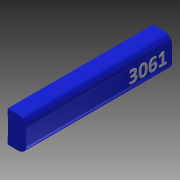
# Autodesk Inventor part: Bumper Cover Part1 (26x28 robot)
Saved by Autodesk Inventor 2013 (Build 170138000, 138)
## iProperties
Created: 2013-01-06
Part Number: Bumper Cover Part1 (26x28 robot)
Material: Generic
Document SubType Name: Modeling
Designer: Moses
Density: 1 g/cm^3
Mass: 433.452 g
Surface Area: 5427.61 cm^2
Volume: 433.452 cm^3
Author: Moses
Autodesk Inventor part; units mm, degrees
ref_plane "YZ Plane" through (0, 0, 0) normal (1, 0, 0) x (0, 1, 0)
ref_plane "XZ Plane" through (0, 0, 0) normal (0, 1, 0) x (-1, 0, 0)
ref_plane "XY Plane" through (0, 0, 0) normal (0, 0, 1) x (1, 0, 0)
sketch "Sketch1" plane through (0, 0, 0) normal (0, 0, 1) x (1, 0, 0)
  line L0 (-6.35, 63.5) -> (-6.35, -63.5) construction
  line L1 (6.35, 63.5) -> (-6.35, 63.5) construction
  line L2 (-6.35, -63.5) -> (6.35, -63.5) construction
  circle A0 centre (38.1, -31.75) radius 31.75 construction
  circle A1 centre (38.1, 31.75) radius 31.75 construction
  line L3 (6.35, 63.5) -> (38.1, 63.5) construction
  line L4 (69.85, 31.75) -> (69.85, -31.75) construction
  line L5 (6.35, -63.5) -> (38.1, -63.5) construction
  line L6 (38.1, 65.0875) -> (-7.9375, 65.0875)
  line L7 (-7.9375, -65.0875) -> (38.1, -65.0875)
  arc A2 (38.1, -65.0875) -> (71.4375, -31.75) centre (38.1, -31.75) ccw
  arc A3 (71.4375, 31.75) -> (38.1, 65.0875) centre (38.1, 31.75) ccw
  line L8 (71.4375, 31.75) -> (71.4375, -31.75)
  line L9 (38.1, 65.0875) -> (38.1, 63.5) construction
  arc A4 (69.85, 31.75) -> (38.1, 63.5) centre (38.1, 31.75) ccw
  arc A5 (38.1, -63.5) -> (69.85, -31.75) centre (38.1, -31.75) ccw
  line L10 (38.1, 63.5) -> (-6.35, 63.5)
  line L11 (38.1, -63.5) -> (-6.35, -63.5)
  line L12 (69.85, 31.75) -> (69.85, -31.75)
  line L13 (-6.35, 63.5) -> (-6.35, 38.1)
  line L14 (-6.35, 38.1) -> (-7.9375, 38.1)
  line L15 (-7.9375, 38.1) -> (-7.9375, 65.0875)
  line L16 (-7.9375, -65.0875) -> (-7.9375, -38.1)
  line L17 (-7.9375, -38.1) -> (-6.35, -38.1)
  line L18 (-6.35, -63.5) -> (-6.35, -38.1)
  line L19 (-6.35, 38.1) -> (-6.35, -38.1)
  point P0 (0, 0)
  point P1 (38.1, 64.2937)
  dimension "d3" = 25.4
  dimension "d5" = 1.5875
  dimension "d6" = 1.5875
  dimension "d7" = 25.4
  dimension "d9" = 1.5875
  constraints: 34 end point, 14 tangent, 12 point on circle, 6 perpendicular, 4 centre point, 3 collinear, 3 parallel, 2 coincident, 2 point on line, 1 concentric, 1 midpoint, 1 vertical
  measures "d3" distance of L0.start L13.end
  measures "d5" distance between parallel lines of L0 L15
  measures "d6" distance between parallel lines of L0 L16
  measures "d7" distance of L0.end L17.end
  measures "d9" distance of L6.start L3.end
extrude "Extrusion1" add sketch "Sketch1" along normal blind 1.5875
extrude "Extrusion2" add sketch "Sketch1" against normal blind 606.425 contours A3 L8 A2 L7 L16 L17 L18 L11 A5 L12 A4 L10 L13 L14 L15 L6
sketch "Sketch2" plane through (0, 0, -606.425) normal (0, 0, -1) x (-1, 0, 0)
  line L0 (-38.1, 63.5) -> (6.35, 63.5) projected
  line L1 (6.35, 63.5) -> (6.35, 38.1) projected
  line L2 (6.35, 38.1) -> (7.9375, 38.1) projected
  line L3 (7.9375, 38.1) -> (7.9375, 65.0875) projected
  line L4 (7.9375, 65.0875) -> (-38.1, 65.0875) projected
  arc A0 (-38.1, 65.0875) -> (-71.4375, 31.75) centre (-38.1, 31.75) ccw projected
  line L5 (-71.4375, 31.75) -> (-71.4375, -31.75) projected
  arc A1 (-71.4375, -31.75) -> (-38.1, -65.0875) centre (-38.1, -31.75) ccw projected
  line L6 (-38.1, -65.0875) -> (7.9375, -65.0875) projected
  line L7 (7.9375, -65.0875) -> (7.9375, -38.1) projected
  line L8 (7.9375, -38.1) -> (6.35, -38.1) projected
  line L9 (6.35, -38.1) -> (6.35, -63.5) projected
  line L10 (6.35, -63.5) -> (-38.1, -63.5) projected
  arc A2 (-69.85, -31.75) -> (-38.1, -63.5) centre (-38.1, -31.75) ccw projected
  line L11 (-69.85, -31.75) -> (-69.85, 31.75) projected
  arc A3 (-38.1, 63.5) -> (-69.85, 31.75) centre (-38.1, 31.75) ccw projected
  line L12 (6.35, 38.1) -> (6.35, -38.1)
  point P0 (0, 0)
  constraints: 2 end point, 1 parallel
extrude "Extrusion3" add sketch "Sketch2" along normal blind 1.5875
sketch "Sketch3" plane through (71.4375, -31.75, 1.5875) normal (1, 0, 0) x (0, 0, -1)
  line L0 (0, 0) -> (0, 63.5) projected
  line L1 (609.6, 63.5) -> (609.6, 0) projected
  line L2 (431.8, 63.5) -> (584.2, 63.5) construction
  line L3 (584.2, 63.5) -> (584.2, 0) construction
  line L4 (584.2, 0) -> (431.8, 0) construction
  line L5 (431.8, 0) -> (431.8, 63.5) construction
  line L6 (609.6, 31.75) -> (0, 31.75) construction
  spline S0 degree 2 poles (464.0687, 21.2561) (464.0687, 17.4878) (461.1591, 11.6208) (456.0075, 7.614) (448.8049, 5.563) (444.5596, 5.563) knots 0 0 0 1 2 3 4 4 4
  spline S1 degree 2 poles (444.5596, 5.563) (441.9839, 5.563) (437.4524, 6.3262) (433.9703, 7.3755) (431.6808, 8.568) (431.013, 9.1881) (430.6314, 9.999) (430.3452, 11.0484) (430.2498, 12.6225) (430.2498, 13.7673) knots 0 0 0 1 2 3 4 5 6 7 8 8 8
  spline S2 degree 2 poles (430.2498, 13.7673) (430.2498, 15.6753) (430.8699, 17.1062) (431.49, 17.1062) knots 0 0 0 1 2 2 2
  spline S3 degree 2 poles (431.49, 17.1062) (431.8716, 17.1062) (433.8272, 16.0569) (436.7846, 14.8167) (440.7914, 13.7673) (443.3194, 13.7673) knots 0 0 0 1 2 3 4 4 4
  spline S4 degree 2 poles (443.3194, 13.7673) (445.4659, 13.7673) (448.7572, 14.769) (451.0468, 16.6293) (452.1915, 19.2527) (452.1915, 20.8268) knots 0 0 0 1 2 3 4 4 4
  spline S5 degree 2 poles (452.1915, 20.8268) (452.1915, 22.5917) (450.8083, 25.406) (448.1371, 27.4093) (444.0349, 28.5064) (441.2207, 28.5064) knots 0 0 0 1 2 3 4 4 4
  line L7 (441.2207, 28.5064) -> (436.8323, 28.5064)
  spline S6 degree 2 poles (436.8323, 28.5064) (436.3553, 28.5064) (435.6398, 28.7926) (435.1628, 29.6512) (434.972, 31.1776) (434.972, 32.3701) knots 0 0 0 1 2 3 4 4 4
  spline S7 degree 2 poles (434.972, 32.3701) (434.972, 33.5149) (435.1628, 34.9459) (435.5921, 35.7091) (436.2599, 36.043) (436.7369, 36.043) knots 0 0 0 1 2 3 4 4 4
  line L8 (436.7369, 36.043) -> (441.173, 36.043)
  spline S8 degree 2 poles (441.173, 36.043) (443.4625, 36.043) (446.9923, 37.0923) (449.3773, 39.048) (450.6175, 41.8146) (450.6175, 43.5318) knots 0 0 0 1 2 3 4 4 4
  spline S9 degree 2 poles (450.6175, 43.5318) (450.6175, 44.8197) (449.7589, 47.1092) (448.0894, 48.7787) (445.4182, 49.7804) (443.6056, 49.7804) knots 0 0 0 1 2 3 4 4 4
  spline S10 degree 2 poles (443.6056, 49.7804) (441.5546, 49.7804) (437.9771, 48.5879) (435.1151, 47.1092) (433.1117, 45.8691) (432.6347, 45.8691) knots 0 0 0 1 2 3 4 4 4
  spline S11 degree 2 poles (432.6347, 45.8691) (432.3485, 45.8691) (431.8716, 46.1553) (431.5377, 46.9185) (431.3946, 48.3971) (431.3946, 49.5896) knots 0 0 0 1 2 3 4 4 4
  spline S12 degree 2 poles (431.3946, 49.5896) (431.3946, 50.5436) (431.49, 51.8315) (431.7285, 52.6901) (432.0623, 53.3102) (432.8255, 54.0734) (435.2582, 55.5521) (438.9311, 56.9831) (443.7487, 57.937) (446.563, 57.937) knots 0 0 0 1 2 3 4 5 6 7 8 8 8
  spline S13 degree 2 poles (446.563, 57.937) (450.2359, 57.937) (455.9121, 56.2199) (459.7758, 52.9763) (461.7792, 48.254) (461.7792, 45.249) knots 0 0 0 1 2 3 4 4 4
  spline S14 degree 2 poles (461.7792, 45.249) (461.7792, 42.9594) (460.5867, 39.0003) (458.3448, 35.8522) (454.9104, 33.658) (452.7162, 33.1333) knots 0 0 0 1 2 3 4 4 4
  line L9 (452.7162, 33.1333) -> (452.7162, 32.9902)
  spline S15 degree 2 poles (452.7162, 32.9902) (455.3397, 32.704) (459.585, 30.6052) (462.4946, 27.5047) (464.0687, 23.5457) (464.0687, 21.2561) knots 0 0 0 1 2 3 4 4 4
  spline S16 degree 2 poles (505.8535, 31.9408) (505.8535, 25.883) (503.8978, 16.1046) (499.4618, 9.2358) (492.4023, 5.563) (487.2984, 5.563) knots 0 0 0 1 2 3 4 4 4
  spline S17 degree 2 poles (487.2984, 5.563) (482.0992, 5.563) (475.2781, 9.1404) (471.3191, 15.8184) (469.6973, 25.4537) (469.6973, 31.5592) knots 0 0 0 1 2 3 4 4 4
  spline S18 degree 2 poles (469.6973, 31.5592) (469.6973, 37.5693) (471.7007, 47.3954) (476.089, 54.2642) (483.1962, 57.937) (488.2524, 57.937) knots 0 0 0 1 2 3 4 4 4
  spline S19 degree 2 poles (488.2524, 57.937) (493.4516, 57.937) (500.3204, 54.3596) (504.2794, 47.6816) (505.8535, 38.0463) (505.8535, 31.9408) knots 0 0 0 1 2 3 4 4 4
  spline S20 degree 2 poles (495.5027, 31.4638) (495.5027, 35.0413) (495.1211, 40.5744) (494.3102, 44.6289) (493.07, 47.4431) (491.3529, 49.1126) (489.1587, 49.8281) (487.8231, 49.8281) knots 0 0 0 1 2 3 4 5 6 6 6
  spline S21 degree 2 poles (487.8231, 49.8281) (485.5335, 49.8281) (482.5285, 47.5862) (480.7636, 43.1502) (480.0481, 36.4723) (480.0481, 32.0839) knots 0 0 0 1 2 3 4 4 4
  spline S22 degree 2 poles (480.0481, 32.0839) (480.0481, 26.6462) (480.9067, 19.5866) (482.7669, 15.3891) (485.6289, 13.7196) (487.68, 13.7196) knots 0 0 0 1 2 3 4 4 4
  spline S23 degree 2 poles (487.68, 13.7196) (489.2064, 13.7196) (491.5437, 14.7213) (493.3085, 16.6769) (494.501, 19.6343) (495.2165, 23.5457) (495.5027, 28.4587) (495.5027, 31.4638) knots 0 0 0 1 2 3 4 5 6 6 6
  spline S24 degree 2 poles (546.1596, 23.3549) (546.1596, 19.5389) (543.8223, 13.0041) (539.2909, 8.2818) (532.613, 5.563) (528.2723, 5.563) knots 0 0 0 1 2 3 4 4 4
  spline S25 degree 2 poles (528.2723, 5.563) (524.7902, 5.563) (519.5433, 7.1847) (515.7273, 10.1898) (513.2946, 14.4828) (511.816, 19.8728) (511.2913, 26.2169) (511.2913, 29.7466) knots 0 0 0 1 2 3 4 5 6 6 6
  spline S26 degree 2 poles (511.2913, 29.7466) (511.2913, 32.704) (511.8637, 39.1911) (513.5808, 45.4398) (516.6336, 51.116) (521.4036, 55.409) (528.2723, 57.8893) (532.9469, 57.8893) knots 0 0 0 1 2 3 4 5 6 6 6
  spline S27 degree 2 poles (532.9469, 57.8893) (534.4255, 57.8893) (537.4783, 57.5554) (540.0541, 56.9831) (541.819, 56.2676) (542.4391, 55.7906) (542.7253, 55.1705) (542.9161, 54.4073) (543.0115, 53.3102) (543.0115, 52.547) knots 0 0 0 1 2 3 4 5 6 7 8 8 8
  spline S28 degree 2 poles (543.0115, 52.547) (543.0115, 51.3068) (542.9161, 49.685) (542.5822, 48.8264) (542.0098, 48.3971) (541.6282, 48.3971) knots 0 0 0 1 2 3 4 4 4
  spline S29 degree 2 poles (541.6282, 48.3971) (541.1512, 48.3971) (539.6725, 48.9218) (537.5737, 49.5419) (534.7117, 50.0189) (532.8515, 50.0189) knots 0 0 0 1 2 3 4 4 4
  spline S30 degree 2 poles (532.8515, 50.0189) (529.6556, 50.0189) (525.2672, 47.6816) (522.5484, 43.6749) (521.3082, 38.3802) (521.2605, 35.4229) knots 0 0 0 1 2 3 4 4 4
  spline S31 degree 2 poles (521.2605, 35.4229) (522.1191, 35.9476) (524.3609, 37.0446) (526.9844, 37.8078) (529.9895, 38.3325) (531.7544, 38.3325) knots 0 0 0 1 2 3 4 4 4
  spline S32 degree 2 poles (531.7544, 38.3325) (535.5703, 38.3325) (541.0558, 36.2338) (544.5378, 32.3224) (546.1596, 26.7416) (546.1596, 23.3549) knots 0 0 0 1 2 3 4 4 4
  spline S33 degree 2 poles (536.095, 22.4009) (536.095, 24.3566) (535.3795, 27.4093) (533.8054, 29.4604) (531.2297, 30.5098) (529.4171, 30.5098) knots 0 0 0 1 2 3 4 4 4
  spline S34 degree 2 poles (529.4171, 30.5098) (528.32, 30.5098) (526.1735, 30.1282) (524.1701, 29.4127) (522.2622, 28.4587) (521.4513, 27.8863) knots 0 0 0 1 2 3 4 4 4
  spline S35 degree 2 poles (521.4513, 27.8863) (521.4513, 23.7365) (522.4053, 18.1079) (524.2178, 14.8644) (527.0321, 13.4811) (528.8447, 13.4811) knots 0 0 0 1 2 3 4 4 4
  spline S36 degree 2 poles (528.8447, 13.4811) (530.6573, 13.4811) (533.3761, 14.8167) (535.141, 17.2493) (536.095, 20.4929) (536.095, 22.4009) knots 0 0 0 1 2 3 4 4 4
  spline S37 degree 2 poles (585.464, 10.3806) (585.464, 9.2835) (585.2255, 7.7571) (584.7962, 6.8508) (584.2715, 6.4693) (583.89, 6.4693) knots 0 0 0 1 2 3 4 4 4
  line L10 (583.89, 6.4693) -> (555.9857, 6.4693)
  spline S38 degree 2 poles (555.9857, 6.4693) (555.6518, 6.4693) (555.1271, 6.8508) (554.6978, 7.7571) (554.4593, 9.2835) (554.4593, 10.3806) knots 0 0 0 1 2 3 4 4 4
  spline S39 degree 2 poles (554.4593, 10.3806) (554.4593, 11.4777) (554.6501, 13.0041) (555.0794, 13.9581) (555.6518, 14.3874) (555.9857, 14.3874) knots 0 0 0 1 2 3 4 4 4
  line L11 (555.9857, 14.3874) -> (565.3825, 14.3874)
  line L12 (565.3825, 14.3874) -> (565.3825, 47.3477)
  line L13 (565.3825, 47.3477) -> (557.2259, 42.864)
  spline S40 degree 2 poles (557.2259, 42.864) (556.3673, 42.4347) (555.2225, 42.2439) (554.5547, 42.9117) (554.3162, 44.5335) (554.3162, 46.0122) knots 0 0 0 1 2 3 4 4 4
  spline S41 degree 2 poles (554.3162, 46.0122) (554.3162, 46.9662) (554.4116, 48.1586) (554.6978, 49.0172) (555.2702, 49.5896) (555.7472, 49.8758) knots 0 0 0 1 2 3 4 4 4
  line L14 (555.7472, 49.8758) -> (566.575, 56.8877)
  spline S42 degree 2 poles (566.575, 56.8877) (566.8135, 57.0785) (567.3859, 57.2692) (568.3399, 57.3646) (569.8663, 57.4123) (571.0588, 57.4123) knots 0 0 0 1 2 3 4 4 4
  spline S43 degree 2 poles (571.0588, 57.4123) (572.5375, 57.4123) (574.3977, 57.3169) (575.304, 57.0308) (575.6379, 56.5538) (575.6379, 56.2199) knots 0 0 0 1 2 3 4 4 4
  line L15 (575.6379, 56.2199) -> (575.6379, 14.3874)
  line L16 (575.6379, 14.3874) -> (583.89, 14.3874)
  spline S44 degree 2 poles (583.89, 14.3874) (584.2715, 14.3874) (584.8439, 13.9581) (585.2732, 13.0041) (585.464, 11.4777) (585.464, 10.3806) knots 0 0 0 1 2 3 4 4 4
  point P0 (1.5875, 31.75)
  point P1 (584.2, 31.75)
  dimension "d41" = 25.4
  dimension "d42" = 152.4
  constraints: 3 midpoint, 2 end point, 2 point on line, 2 other
  measures "d41" distance between parallel lines of L1 L3
  measures "d42" distance between parallel lines of L3 L5
extrude "Extrusion5" add sketch "Sketch3" along normal blind 1.5875
body "Solid1"
